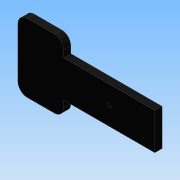
# Autodesk Inventor part: PCB_slit_circle_1.5mm
Saved by Autodesk Inventor 2016 (Build 200138000, 138)
## iProperties
Created: 2015-08-14
Part Number: PCB_slit_circle_1.5mm
Material: Generic
Document SubType Name: Modeling
Designer: Openlab
Density: 1 g/cm^3
Appearance: Glossy - Black
Author: Openlab
Autodesk Inventor part; units mm, degrees
ref_plane "YZ Plane" through (0, 0, 0) normal (1, 0, 0) x (0, 1, 0)
ref_plane "XZ Plane" through (0, 0, 0) normal (0, 1, 0) x (-1, 0, 0)
ref_plane "XY Plane" through (0, 0, 0) normal (0, 0, 1) x (1, 0, 0)
sketch "Sketch1" plane through (0, 0, 0) normal (0, 1, 0) x (-1, 0, 0)
  line L0 (0, 0) -> (20, 0)
  line L1 (20, -8) -> (0, -8)
  line L2 (0, -8) -> (0, 0)
  line L3 (20, 0) -> (20, 1.5)
  line L4 (22, 3.5) -> (28, 3.5)
  line L5 (30, 1.5) -> (30, -9.5)
  line L6 (28, -11.5) -> (22, -11.5)
  line L7 (20, -9.5) -> (20, -8)
  line L8 (13.2363, -4) -> (6.6675, -4) construction
  arc A0 (30, 1.5) -> (28, 3.5) centre (28, 1.5) ccw
  arc A1 (22, 3.5) -> (20, 1.5) centre (22, 1.5) ccw
  arc A2 (28, -11.5) -> (30, -9.5) centre (28, -9.5) ccw
  arc A3 (20, -9.5) -> (22, -11.5) centre (22, -9.5) ccw
  line L9 (10, -2.0671) -> (10, -6.5599) construction
  circle A4 centre (10, -4) radius 0.5
  point P0 (30, 3.5)
  point P1 (30, -11.5)
  point P2 (20, -11.5)
  dimension "d0" = 20
  dimension "d1" = 8
  dimension "d2" = 15
  dimension "d3" = 10
  dimension "d4" = 2
  dimension "d5" = 1
  constraints: 20 end point, 9 point on line, 8 point on circle, 8 tangent, 5 centre point, 5 perpendicular, 3 equal radius, 2 horizontal, 2 vertical, 1 parallel, 3 other
  measures "d0" distance of L1.start L1.end
  measures "d1" distance of L0.end L1.start
  measures "d2" distance of point (30, 3.5) point (30, -11.5)
  measures "d3" distance of point (30, -11.5) point (20, -11.5)
  measures "d4" radius of A0
  measures "d5" diameter of A4
extrude "Extrusion1" add sketch "Sketch1" along normal blind 1.6
body "Solid1"
